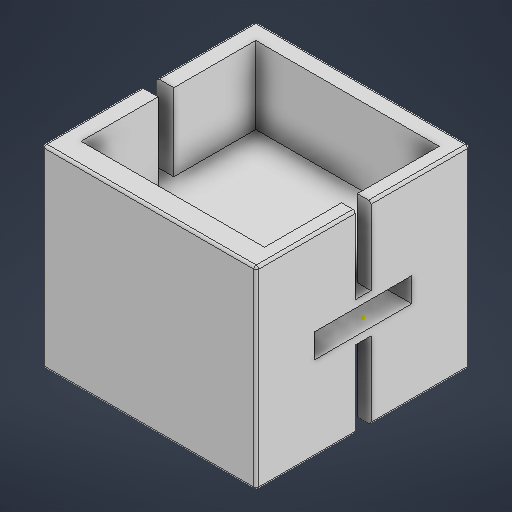
# Autodesk Inventor part: Base_Casing
Saved by Autodesk Inventor 2026.1 (Build 301233000, 233)
## iProperties
Created: 2025-09-05
Part Number: Base_Casing
Material: Generic
Document SubType Name: Modeling
Designer: usman
Density: 1 g/cm^3
Appearance: Default
Author: usman
Autodesk Inventor part; units mm, degrees
ref_plane "YZ Plane" through (0, 0, 0) normal (1, 0, 0) x (0, 1, 0)
ref_plane "XZ Plane" through (0, 0, 0) normal (0, 1, 0) x (-1, 0, 0)
ref_plane "XY Plane" through (0, 0, 0) normal (0, 0, 1) x (1, 0, 0)
sketch "Sketch1" plane through (0, 0, 0) normal (1, 0, 0) x (0, 1, 0)
  line L0 (-39.75, 43.9) -> (39.75, 43.9)
  line L1 (39.75, 43.9) -> (39.75, -43.9)
  line L2 (39.75, -43.9) -> (-39.75, -43.9)
  line L3 (-39.75, -43.9) -> (-39.75, 43.9)
  line L4 (-39.75, 43.9) -> (39.75, -43.9) construction
  line L5 (39.75, 43.9) -> (-39.75, -43.9) construction
  point P0 (0, 0)
  dimension "d0" = 79.5
  dimension "d1" = 87.8
  constraints: 12 end point, 2 midpoint, 2 parallel, 1 horizontal, 1 perpendicular
  measures "d0" distance of L1.end L2.end
  measures "d1" distance of L0.end L1.end
extrude "Extrusion1" add sketch "Sketch1" along normal blind 88
sketch "Sketch2" plane through (88, 0, 0) normal (1, 0, 0) x (0, 0, -1)
  line L0 (-20, -5) -> (20, -5)
  line L1 (20, -5) -> (20, 5)
  line L2 (20, 5) -> (-20, 5)
  line L3 (-20, 5) -> (-20, -5)
  line L4 (-20, -5) -> (20, 5) construction
  line L5 (20, -5) -> (-20, 5) construction
  point P0 (0, 0)
  dimension "d4" = 10
  dimension "d5" = 40
  constraints: 12 end point, 2 midpoint, 2 parallel, 1 horizontal, 1 perpendicular
  measures "d4" distance of L0.end L1.end
  measures "d5" distance of L1.end L2.end
extrude "Extrusion2" cut sketch "Sketch2" against normal through all
sketch "Sketch3" plane through (88, 0, 0) normal (1, 0, 0) x (0, 0, -1)
  point P0 (0, 0)
sketch "Sketch4" plane through (0, 39.75, 43.9) normal (0, 1, 0) x (1, 0, 0)
  line L0 (82.3836, 9.0103) -> (7, 9.0103)
  line L1 (7, 9.0103) -> (7, 80.8)
  line L2 (7, 80.8) -> (82.3836, 80.8)
  line L3 (82.3836, 80.8) -> (82.3836, 9.0103)
  line L4 (82.3836, 9.0103) -> (7, 80.8) construction
  line L5 (7, 9.0103) -> (82.3836, 80.8) construction
  line L6 (0, 87.8) -> (0, 0) projected
  line L7 (0, 87.8) -> (88, 87.8) projected
  point P0 (0, 43.9)
  point P1 (44.6918, 44.9051)
  dimension "d8" = 7
  dimension "d9" = 7
  constraints: 12 end point, 2 midpoint, 2 parallel, 1 horizontal, 1 perpendicular
  measures "d8" distance between parallel lines of L6 L1
  measures "d9" distance between parallel lines of L7 L2
extrude "Extrusion3" cut sketch "Sketch4" against normal blind 31.7
mirror "Mirror1" about plane through (0, 0, 0) normal (0, 1, 0) of "Extrusion3"
sketch "Sketch5" plane through (0, 0, 0) normal (-1, 0, 0) x (0, 0, 1)
  line L0 (-43.9, 39.75) -> (43.9, 39.75) projected
  line L1 (-3.25, 8.05) -> (3.25, 8.05)
  line L2 (3.25, 8.05) -> (3.25, 39.75)
  line L3 (3.25, 39.75) -> (-3.25, 39.75)
  line L4 (-3.25, 39.75) -> (-3.25, 8.05)
  line L5 (-3.25, 8.05) -> (3.25, 39.75) construction
  line L6 (3.25, 8.05) -> (-3.25, 39.75) construction
  point P0 (0, 0)
  point P1 (0, 23.9)
  point P2 (-3.25, 39.75)
  dimension "d12" = 3.25
  dimension "d13" = 31.7
  constraints: 12 end point, 2 midpoint, 2 parallel, 1 horizontal, 1 perpendicular, 1 point on line
  measures "d12" distance from line of point (0, 23.9) L2
  measures "d13" distance of L1.end L2.end
extrude "Extrusion4" cut sketch "Sketch5" against normal through all
mirror "Mirror2" about plane through (0, 0, 0) normal (0, 1, 0) of "Extrusion4"
sketch "Sketch6" plane through (0, 0, 0) normal (-1, 0, 0) x (0, 0, 1)
  line L0 (-43.5136, 38.271) -> (-4.0193, 38.271) construction
  line L1 (-4.0193, 38.271) -> (-4.0193, 7.5144) construction
  line L2 (-4.0193, 7.5144) -> (-43.5136, 7.5144) construction
  line L3 (-43.5136, 7.5144) -> (-43.5136, 38.271) construction
  line L4 (-32.9155, 25.9076) -> (-32.9155, 32.0036)
  line L5 (-32.9155, 32.0036) -> (-31.9606, 32.0036)
  spline S0 degree 2 poles (-31.9606, 32.0036) (-31.1264, 32.0036) (-30.7394, 31.898) knots 0 0 0 1 1 1
  spline S1 degree 2 poles (-30.7394, 31.898) (-30.1967, 31.7523) (-29.5484, 30.9633) (-29.5484, 30.4306) knots 0 0 0 1 2 2 2
  spline S2 degree 2 poles (-29.5484, 30.4306) (-29.5484, 30.0788) (-29.8398, 29.5109) (-30.1715, 29.2647) knots 0 0 0 1 2 2 2
  spline S3 degree 2 poles (-30.1715, 29.2647) (-29.6137, 29.0033) (-29.1011, 28.2193) (-29.1011, 27.6866) knots 0 0 0 1 2 2 2
  spline S4 degree 2 poles (-29.1011, 27.6866) (-29.1011, 27.169) (-29.6338, 26.3247) (-30.468, 25.9076) (-31.2068, 25.9076) knots 0 0 0 1 2 3 3 3
  line L6 (-31.2068, 25.9076) -> (-32.9155, 25.9076)
  line L7 (-31.7546, 28.5762) -> (-31.7546, 27.0132)
  line L8 (-31.7546, 27.0132) -> (-31.4631, 27.0132)
  spline S5 degree 2 poles (-31.4631, 27.0132) (-30.7444, 27.0132) (-30.2419, 27.3801) (-30.2419, 27.7268) knots 0 0 0 1 2 2 2
  spline S6 degree 2 poles (-30.2419, 27.7268) (-30.2419, 28.1188) (-30.8299, 28.5762) (-31.5134, 28.5762) knots 0 0 0 1 2 2 2
  line L9 (-31.5134, 28.5762) -> (-31.7546, 28.5762)
  line L10 (-31.7546, 30.898) -> (-31.7546, 29.6114)
  line L11 (-31.7546, 29.6114) -> (-31.5033, 29.6114)
  spline S7 degree 2 poles (-31.5033, 29.6114) (-31.0812, 29.6114) (-30.6691, 29.9682) (-30.6691, 30.2748) knots 0 0 0 1 2 2 2
  spline S8 degree 2 poles (-30.6691, 30.2748) (-30.6691, 30.5612) (-31.056, 30.898) (-31.4581, 30.898) knots 0 0 0 1 2 2 2
  line L12 (-31.4581, 30.898) -> (-31.7546, 30.898)
  line L13 (-24.7892, 30.4155) -> (-23.6584, 30.4155)
  line L14 (-23.6584, 30.4155) -> (-23.6584, 25.9076)
  line L15 (-23.6584, 25.9076) -> (-24.7892, 25.9076)
  line L16 (-24.7892, 25.9076) -> (-24.7892, 26.385)
  spline S9 degree 2 poles (-24.7892, 26.385) (-25.1208, 26.0684) (-25.7842, 25.792) (-26.1762, 25.792) knots 0 0 0 1 2 2 2
  spline S10 degree 2 poles (-26.1762, 25.792) (-27.0456, 25.792) (-28.3221, 27.1489) (-28.3221, 28.154) knots 0 0 0 1 2 2 2
  spline S11 degree 2 poles (-28.3221, 28.154) (-28.3221, 29.1993) (-27.0909, 30.5311) (-26.2064, 30.5311) knots 0 0 0 1 2 2 2
  spline S12 degree 2 poles (-26.2064, 30.5311) (-25.8043, 30.5311) (-25.0907, 30.2245) (-24.7892, 29.918) knots 0 0 0 1 2 2 2
  line L17 (-24.7892, 29.918) -> (-24.7892, 30.4155)
  spline S13 degree 2 poles (-25.9802, 29.4858) (-26.5029, 29.4858) (-27.1964, 28.747) (-27.1964, 28.1641) knots 0 0 0 1 2 2 2
  spline S14 degree 2 poles (-27.1964, 28.1641) (-27.1964, 27.5811) (-26.4878, 26.8273) (-25.9752, 26.8273) knots 0 0 0 1 2 2 2
  spline S15 degree 2 poles (-25.9752, 26.8273) (-25.4425, 26.8273) (-24.7389, 27.571) (-24.7389, 28.1691) knots 0 0 0 1 2 2 2
  spline S16 degree 2 poles (-24.7389, 28.1691) (-24.7389, 28.7571) (-25.4425, 29.4858) (-25.9802, 29.4858) knots 0 0 0 1 2 2 2
  line L18 (-19.7586, 29.7823) -> (-20.4571, 29.0837)
  spline S17 degree 2 poles (-20.4571, 29.0837) (-20.8793, 29.5059) (-21.226, 29.5059) knots 0 0 0 1 1 1
  spline S18 degree 2 poles (-21.226, 29.5059) (-21.417, 29.5059) (-21.6331, 29.3451) (-21.6331, 29.2244) knots 0 0 0 1 2 2 2
  spline S19 degree 2 poles (-21.6331, 29.2244) (-21.6331, 29.134) (-21.4974, 28.9782) (-21.226, 28.8475) knots 0 0 0 1 2 2 2
  line L19 (-21.226, 28.8475) -> (-20.8139, 28.6415)
  spline S20 degree 2 poles (-20.8139, 28.6415) (-20.1606, 28.3198) (-19.6731, 27.6464) (-19.6731, 27.1941) knots 0 0 0 1 2 2 2
  spline S21 degree 2 poles (-19.6731, 27.1941) (-19.6731, 26.5961) (-20.5526, 25.792) (-21.2964, 25.792) knots 0 0 0 1 2 2 2
  spline S22 degree 2 poles (-21.2964, 25.792) (-22.2814, 25.792) (-22.8694, 26.5609) knots 0 0 0 1 1 1
  line L20 (-22.8694, 26.5609) -> (-22.1759, 27.3198)
  spline S23 degree 2 poles (-22.1759, 27.3198) (-21.9748, 27.0886) (-21.4421, 26.8021) (-21.2361, 26.8021) knots 0 0 0 1 2 2 2
  spline S24 degree 2 poles (-21.2361, 26.8021) (-21.0099, 26.8021) (-20.7386, 27.0182) (-20.7386, 27.1589) knots 0 0 0 1 2 2 2
  spline S25 degree 2 poles (-20.7386, 27.1589) (-20.7386, 27.4203) (-21.2311, 27.6665) knots 0 0 0 1 1 1
  line L21 (-21.2311, 27.6665) -> (-21.613, 27.8575)
  spline S26 degree 2 poles (-21.613, 27.8575) (-22.7036, 28.4103) (-22.7036, 29.2395) knots 0 0 0 1 1 1
  spline S27 degree 2 poles (-22.7036, 29.2395) (-22.7036, 29.7722) (-21.8794, 30.5311) (-21.2411, 30.5311) knots 0 0 0 1 2 2 2
  spline S28 degree 2 poles (-21.2411, 30.5311) (-20.7989, 30.5311) (-20.0249, 30.1441) (-19.7586, 29.7823) knots 0 0 0 1 2 2 2
  line L22 (-14.2656, 27.8374) -> (-17.8941, 27.8374)
  spline S29 degree 2 poles (-17.8941, 27.8374) (-17.8137, 27.3549) (-17.1302, 26.7871) (-16.6025, 26.7871) knots 0 0 0 1 2 2 2
  spline S30 degree 2 poles (-16.6025, 26.7871) (-15.9693, 26.7871) (-15.512, 27.2293) knots 0 0 0 1 1 1
  line L23 (-15.512, 27.2293) -> (-14.5621, 26.782)
  spline S31 degree 2 poles (-14.5621, 26.782) (-14.919, 26.2795) (-15.914, 25.792) (-16.5975, 25.792) knots 0 0 0 1 2 2 2
  spline S32 degree 2 poles (-16.5975, 25.792) (-17.6579, 25.792) (-18.9897, 27.1288) (-18.9897, 28.1389) knots 0 0 0 1 2 2 2
  spline S33 degree 2 poles (-18.9897, 28.1389) (-18.9897, 29.1692) (-17.6579, 30.5311) (-16.6578, 30.5311) knots 0 0 0 1 2 2 2
  spline S34 degree 2 poles (-16.6578, 30.5311) (-15.5924, 30.5311) (-14.2606, 29.1692) (-14.2606, 28.0535) knots 0 0 0 1 2 2 2
  line L24 (-14.2606, 28.0535) -> (-14.2656, 27.8374)
  spline S35 degree 2 poles (-15.3964, 28.7269) (-15.507, 29.1038) (-16.1653, 29.5712) (-16.6025, 29.5712) knots 0 0 0 1 2 2 2
  spline S36 degree 2 poles (-16.6025, 29.5712) (-17.0749, 29.5712) (-17.4317, 29.3099) knots 0 0 0 1 1 1
  spline S37 degree 2 poles (-17.4317, 29.3099) (-17.6529, 29.144) (-17.8438, 28.7269) knots 0 0 0 1 1 1
  line L25 (-17.8438, 28.7269) -> (-15.3964, 28.7269)
  line L26 (-38.4386, 21.6418) -> (-37.3128, 21.6418)
  line L27 (-37.3128, 21.6418) -> (-35.8956, 17.3901)
  line L28 (-35.8956, 17.3901) -> (-34.4684, 21.6418)
  line L29 (-34.4684, 21.6418) -> (-33.3427, 21.6418)
  line L30 (-33.3427, 21.6418) -> (-32.3225, 15.5458)
  line L31 (-32.3225, 15.5458) -> (-33.4432, 15.5458)
  line L32 (-33.4432, 15.5458) -> (-34.0915, 19.3953)
  line L33 (-34.0915, 19.3953) -> (-35.3881, 15.5458)
  line L34 (-35.3881, 15.5458) -> (-36.4133, 15.5458)
  line L35 (-36.4133, 15.5458) -> (-37.6948, 19.3953)
  line L36 (-37.6948, 19.3953) -> (-38.3632, 15.5458)
  line L37 (-38.3632, 15.5458) -> (-39.4939, 15.5458)
  line L38 (-39.4939, 15.5458) -> (-38.4386, 21.6418)
  line L39 (-28.1864, 20.0537) -> (-27.0557, 20.0537)
  line L40 (-27.0557, 20.0537) -> (-27.0557, 15.5458)
  line L41 (-27.0557, 15.5458) -> (-28.1864, 15.5458)
  line L42 (-28.1864, 15.5458) -> (-28.1864, 16.0232)
  spline S38 degree 2 poles (-28.1864, 16.0232) (-28.5181, 15.7066) (-29.1815, 15.4302) (-29.5735, 15.4302) knots 0 0 0 1 2 2 2
  spline S39 degree 2 poles (-29.5735, 15.4302) (-30.4429, 15.4302) (-31.7194, 16.7871) (-31.7194, 17.7922) knots 0 0 0 1 2 2 2
  spline S40 degree 2 poles (-31.7194, 17.7922) (-31.7194, 18.8375) (-30.4881, 20.1693) (-29.6036, 20.1693) knots 0 0 0 1 2 2 2
  spline S41 degree 2 poles (-29.6036, 20.1693) (-29.2016, 20.1693) (-28.488, 19.8627) (-28.1864, 19.5562) knots 0 0 0 1 2 2 2
  line L43 (-28.1864, 19.5562) -> (-28.1864, 20.0537)
  spline S42 degree 2 poles (-29.3775, 19.124) (-29.9001, 19.124) (-30.5937, 18.3852) (-30.5937, 17.8022) knots 0 0 0 1 2 2 2
  spline S43 degree 2 poles (-30.5937, 17.8022) (-30.5937, 17.2193) (-29.8851, 16.4654) (-29.3725, 16.4654) knots 0 0 0 1 2 2 2
  spline S44 degree 2 poles (-29.3725, 16.4654) (-28.8398, 16.4654) (-28.1362, 17.2092) (-28.1362, 17.8073) knots 0 0 0 1 2 2 2
  spline S45 degree 2 poles (-28.1362, 17.8073) (-28.1362, 18.3953) (-28.8398, 19.124) (-29.3775, 19.124) knots 0 0 0 1 2 2 2
  line L44 (-22.5829, 20.0537) -> (-21.4522, 20.0537)
  line L45 (-21.4522, 20.0537) -> (-21.4522, 16.1941)
  spline S46 degree 2 poles (-21.4522, 16.1941) (-21.4522, 15.0482) (-21.9145, 14.5105) knots 0 0 0 1 1 1
  spline S47 degree 2 poles (-21.9145, 14.5105) (-22.5277, 13.7818) (-23.774, 13.7818) knots 0 0 0 1 1 1
  spline S48 degree 2 poles (-23.774, 13.7818) (-24.4374, 13.7818) (-25.3369, 14.1135) (-25.9601, 14.7568) (-26.1109, 15.2141) knots 0 0 0 1 2 3 3 3
  line L46 (-26.1109, 15.2141) -> (-24.8645, 15.2141)
  spline S49 degree 2 poles (-24.8645, 15.2141) (-24.6987, 15.0231) (-24.176, 14.8321) (-23.8192, 14.8321) knots 0 0 0 1 2 2 2
  spline S50 degree 2 poles (-23.8192, 14.8321) (-23.3669, 14.8321) (-22.8091, 15.1136) (-22.5829, 15.5608) (-22.5829, 16.1086) knots 0 0 0 1 2 3 3 3
  spline S51 degree 2 poles (-22.5829, 16.1086) (-22.8794, 15.8071) (-23.5328, 15.5458) (-23.9499, 15.5458) knots 0 0 0 1 2 2 2
  spline S52 degree 2 poles (-23.9499, 15.5458) (-24.8545, 15.5458) (-26.1059, 16.8574) (-26.1059, 17.8575) knots 0 0 0 1 2 2 2
  spline S53 degree 2 poles (-26.1059, 17.8575) (-26.1059, 18.933) (-25.4425, 19.5813) knots 0 0 0 1 1 1
  spline S54 degree 2 poles (-25.4425, 19.5813) (-24.8444, 20.1693) (-24.0102, 20.1693) knots 0 0 0 1 1 1
  spline S55 degree 2 poles (-24.0102, 20.1693) (-23.6232, 20.1693) (-22.9297, 19.8828) (-22.5829, 19.5562) knots 0 0 0 1 2 2 2
  line L47 (-22.5829, 19.5562) -> (-22.5829, 20.0537)
  spline S56 degree 2 poles (-23.7489, 19.1139) (-24.2866, 19.1139) (-24.9801, 18.3953) (-24.9801, 17.8525) knots 0 0 0 1 2 2 2
  spline S57 degree 2 poles (-24.9801, 17.8525) (-24.9801, 17.2896) (-24.2665, 16.571) (-23.7288, 16.571) knots 0 0 0 1 2 2 2
  spline S58 degree 2 poles (-23.7288, 16.571) (-23.2061, 16.571) (-22.5226, 17.2746) (-22.5226, 17.8475) knots 0 0 0 1 2 2 2
  spline S59 degree 2 poles (-22.5226, 17.8475) (-22.5226, 18.4103) (-23.2111, 19.1139) (-23.7489, 19.1139) knots 0 0 0 1 2 2 2
  line L48 (-20.3064, 20.0537) -> (-19.1756, 20.0537)
  line L49 (-19.1756, 20.0537) -> (-19.1756, 19.5913)
  spline S60 degree 2 poles (-19.1756, 19.5913) (-18.7886, 19.918) (-18.1655, 20.1693) (-17.8388, 20.1693) knots 0 0 0 1 2 2 2
  spline S61 degree 2 poles (-17.8388, 20.1693) (-17.1654, 20.1693) (-16.698, 19.7019) knots 0 0 0 1 1 1
  spline S62 degree 2 poles (-16.698, 19.7019) (-16.306, 19.3049) (-16.306, 18.5259) knots 0 0 0 1 1 1
  line L50 (-16.306, 18.5259) -> (-16.306, 15.5458)
  line L51 (-16.306, 15.5458) -> (-17.4267, 15.5458)
  line L52 (-17.4267, 15.5458) -> (-17.4267, 17.5208)
  spline S63 degree 2 poles (-17.4267, 17.5208) (-17.4267, 18.3249) (-17.5725, 18.8576) (-17.9293, 19.134) (-18.1956, 19.134) knots 0 0 0 1 2 3 3 3
  spline S64 degree 2 poles (-18.1956, 19.134) (-18.5374, 19.134) (-19.0299, 18.6767) (-19.1254, 18.2696) knots 0 0 0 1 2 2 2
  spline S65 degree 2 poles (-19.1254, 18.2696) (-19.1756, 18.0585) (-19.1756, 17.355) knots 0 0 0 1 1 1
  line L53 (-19.1756, 17.355) -> (-19.1756, 15.5458)
  line L54 (-19.1756, 15.5458) -> (-20.3064, 15.5458)
  line L55 (-20.3064, 15.5458) -> (-20.3064, 20.0537)
  line L56 (-10.6975, 17.4756) -> (-14.3259, 17.4756)
  spline S66 degree 2 poles (-14.3259, 17.4756) (-14.2455, 16.9931) (-13.5621, 16.4252) (-13.0344, 16.4252) knots 0 0 0 1 2 2 2
  spline S67 degree 2 poles (-13.0344, 16.4252) (-12.4012, 16.4252) (-11.9438, 16.8675) knots 0 0 0 1 1 1
  line L57 (-11.9438, 16.8675) -> (-10.994, 16.4202)
  spline S68 degree 2 poles (-10.994, 16.4202) (-11.3508, 15.9177) (-12.3459, 15.4302) (-13.0294, 15.4302) knots 0 0 0 1 2 2 2
  spline S69 degree 2 poles (-13.0294, 15.4302) (-14.0897, 15.4302) (-15.4215, 16.767) (-15.4215, 17.7771) knots 0 0 0 1 2 2 2
  spline S70 degree 2 poles (-15.4215, 17.7771) (-15.4215, 18.8074) (-14.0897, 20.1693) (-13.0897, 20.1693) knots 0 0 0 1 2 2 2
  spline S71 degree 2 poles (-13.0897, 20.1693) (-12.0242, 20.1693) (-10.6925, 18.8074) (-10.6925, 17.6917) knots 0 0 0 1 2 2 2
  line L58 (-10.6925, 17.6917) -> (-10.6975, 17.4756)
  spline S72 degree 2 poles (-11.8282, 18.3651) (-11.9388, 18.742) (-12.5972, 19.2094) (-13.0344, 19.2094) knots 0 0 0 1 2 2 2
  spline S73 degree 2 poles (-13.0344, 19.2094) (-13.5068, 19.2094) (-13.8636, 18.9481) knots 0 0 0 1 1 1
  spline S74 degree 2 poles (-13.8636, 18.9481) (-14.0847, 18.7822) (-14.2757, 18.3651) knots 0 0 0 1 1 1
  line L59 (-14.2757, 18.3651) -> (-11.8282, 18.3651)
  line L60 (-9.6421, 21.7172) -> (-8.5114, 21.7172)
  line L61 (-8.5114, 21.7172) -> (-8.5114, 20.0537)
  line L62 (-8.5114, 20.0537) -> (-7.838, 20.0537)
  line L63 (-7.838, 20.0537) -> (-7.838, 19.0787)
  line L64 (-7.838, 19.0787) -> (-8.5114, 19.0787)
  line L65 (-8.5114, 19.0787) -> (-8.5114, 15.5458)
  line L66 (-8.5114, 15.5458) -> (-9.6421, 15.5458)
  line L67 (-9.6421, 15.5458) -> (-9.6421, 19.0787)
  line L68 (-9.6421, 19.0787) -> (-10.2201, 19.0787)
  line L69 (-10.2201, 19.0787) -> (-10.2201, 20.0537)
  line L70 (-10.2201, 20.0537) -> (-9.6421, 20.0537)
  line L71 (-9.6421, 20.0537) -> (-9.6421, 21.7172)
  point P0 (0, 0)
  dimension "d0" = 79.5
  dimension "d1" = 87.8
  constraints: 2 other
sketch "Sketch7" plane through (0, 0, 0) normal (-1, 0, 0) x (0, 0, 1)
  line L0 (5.4174, 37.9215) -> (42.8146, 37.9215) construction
  line L1 (42.8146, 37.9215) -> (42.8146, 6.8154) construction
  line L2 (42.8146, 6.8154) -> (5.4174, 6.8154) construction
  line L3 (5.4174, 6.8154) -> (5.4174, 37.9215) construction
  line L4 (-40.9304, -8.5629) -> (-3.951, -8.5629) construction
  line L5 (-3.951, -8.5629) -> (-3.951, -37.9215) construction
  line L6 (-3.951, -37.9215) -> (-40.9304, -37.9215) construction
  line L7 (-40.9304, -37.9215) -> (-40.9304, -8.5629) construction
  line L8 (16.0675, 25.0873) -> (15.2584, 24.3133)
  spline S0 degree 2 poles (15.2584, 24.3133) (14.4292, 25.1878) (13.3939, 25.1878) knots 0 0 0 1 1 1
  spline S1 degree 2 poles (13.3939, 25.1878) (12.5195, 25.1878) (11.3234, 23.9967) (11.3234, 23.1223) knots 0 0 0 1 2 2 2
  spline S2 degree 2 poles (11.3234, 23.1223) (11.3234, 22.5142) (11.8511, 21.5694) (12.821, 21.0316) (13.414, 21.0316) knots 0 0 0 1 2 3 3 3
  spline S3 degree 2 poles (13.414, 21.0316) (13.9166, 21.0316) (14.7559, 21.4085) (15.2584, 21.9061) knots 0 0 0 1 2 2 2
  line L9 (15.2584, 21.9061) -> (16.0424, 21.0869)
  spline S4 degree 2 poles (16.0424, 21.0869) (15.369, 20.4235) (14.1679, 19.916) (13.3939, 19.916) knots 0 0 0 1 2 2 2
  spline S5 degree 2 poles (13.3939, 19.916) (11.9717, 19.916) (10.1625, 21.7151) (10.1625, 23.1273) knots 0 0 0 1 2 2 2
  spline S6 degree 2 poles (10.1625, 23.1273) (10.1625, 24.0369) (10.9867, 25.4541) (12.5245, 26.3135) (13.409, 26.3135) knots 0 0 0 1 2 3 3 3
  spline S7 degree 2 poles (13.409, 26.3135) (14.1679, 26.3135) (15.56, 25.6752) (16.0675, 25.0873) knots 0 0 0 1 2 2 2
  line L10 (20.289, 24.5746) -> (21.4198, 24.5746)
  line L11 (21.4198, 24.5746) -> (21.4198, 20.0667)
  line L12 (21.4198, 20.0667) -> (20.289, 20.0667)
  line L13 (20.289, 20.0667) -> (20.289, 20.5442)
  spline S8 degree 2 poles (20.289, 20.5442) (19.9573, 20.2275) (19.2939, 19.9511) (18.9019, 19.9511) knots 0 0 0 1 2 2 2
  spline S9 degree 2 poles (18.9019, 19.9511) (18.0325, 19.9511) (16.756, 21.308) (16.756, 22.3131) knots 0 0 0 1 2 2 2
  spline S10 degree 2 poles (16.756, 22.3131) (16.756, 23.3585) (17.9873, 24.6902) (18.8718, 24.6902) knots 0 0 0 1 2 2 2
  spline S11 degree 2 poles (18.8718, 24.6902) (19.2738, 24.6902) (19.9875, 24.3837) (20.289, 24.0771) knots 0 0 0 1 2 2 2
  line L14 (20.289, 24.0771) -> (20.289, 24.5746)
  spline S12 degree 2 poles (19.0979, 23.6449) (18.5753, 23.6449) (17.8818, 22.9062) (17.8818, 22.3232) knots 0 0 0 1 2 2 2
  spline S13 degree 2 poles (17.8818, 22.3232) (17.8818, 21.7402) (18.5904, 20.9864) (19.103, 20.9864) knots 0 0 0 1 2 2 2
  spline S14 degree 2 poles (19.103, 20.9864) (19.6357, 20.9864) (20.3393, 21.7302) (20.3393, 22.3282) knots 0 0 0 1 2 2 2
  spline S15 degree 2 poles (20.3393, 22.3282) (20.3393, 22.9162) (19.6357, 23.6449) (19.0979, 23.6449) knots 0 0 0 1 2 2 2
  line L15 (25.3196, 23.9414) -> (24.621, 23.2429)
  spline S16 degree 2 poles (24.621, 23.2429) (24.1989, 23.665) (23.8521, 23.665) knots 0 0 0 1 1 1
  spline S17 degree 2 poles (23.8521, 23.665) (23.6612, 23.665) (23.4451, 23.5042) (23.4451, 23.3836) knots 0 0 0 1 2 2 2
  spline S18 degree 2 poles (23.4451, 23.3836) (23.4451, 23.2931) (23.5807, 23.1373) (23.8521, 23.0067) knots 0 0 0 1 2 2 2
  line L16 (23.8521, 23.0067) -> (24.2642, 22.8006)
  spline S19 degree 2 poles (24.2642, 22.8006) (24.9175, 22.479) (25.405, 21.8056) (25.405, 21.3533) knots 0 0 0 1 2 2 2
  spline S20 degree 2 poles (25.405, 21.3533) (25.405, 20.7552) (24.5255, 19.9511) (23.7818, 19.9511) knots 0 0 0 1 2 2 2
  spline S21 degree 2 poles (23.7818, 19.9511) (22.7968, 19.9511) (22.2088, 20.72) knots 0 0 0 1 1 1
  line L17 (22.2088, 20.72) -> (22.9023, 21.4789)
  spline S22 degree 2 poles (22.9023, 21.4789) (23.1033, 21.2477) (23.636, 20.9613) (23.8421, 20.9613) knots 0 0 0 1 2 2 2
  spline S23 degree 2 poles (23.8421, 20.9613) (24.0682, 20.9613) (24.3396, 21.1774) (24.3396, 21.3181) knots 0 0 0 1 2 2 2
  spline S24 degree 2 poles (24.3396, 21.3181) (24.3396, 21.5794) (23.8471, 21.8257) knots 0 0 0 1 1 1
  line L18 (23.8471, 21.8257) -> (23.4652, 22.0166)
  spline S25 degree 2 poles (23.4652, 22.0166) (22.3746, 22.5695) (22.3746, 23.3987) knots 0 0 0 1 1 1
  spline S26 degree 2 poles (22.3746, 23.3987) (22.3746, 23.9314) (23.1988, 24.6902) (23.837, 24.6902) knots 0 0 0 1 2 2 2
  spline S27 degree 2 poles (23.837, 24.6902) (24.2793, 24.6902) (25.0532, 24.3033) (25.3196, 23.9414) knots 0 0 0 1 2 2 2
  line L19 (26.1739, 24.5746) -> (27.3047, 24.5746)
  line L20 (27.3047, 24.5746) -> (27.3047, 20.0667)
  line L21 (27.3047, 20.0667) -> (26.1739, 20.0667)
  line L22 (26.1739, 20.0667) -> (26.1739, 24.5746)
  spline S28 degree 2 poles (26.7368, 26.4341) (27.0333, 26.4341) (27.4605, 26.0019) (27.4605, 25.6953) knots 0 0 0 1 2 2 2
  spline S29 degree 2 poles (27.4605, 25.6953) (27.4605, 25.3938) (27.0383, 24.9666) (26.7468, 24.9666) knots 0 0 0 1 2 2 2
  spline S30 degree 2 poles (26.7468, 24.9666) (26.4453, 24.9666) (26.0181, 25.4039) (26.0181, 25.7104) knots 0 0 0 1 2 2 2
  spline S31 degree 2 poles (26.0181, 25.7104) (26.0181, 26.012) (26.4403, 26.4341) (26.7368, 26.4341) knots 0 0 0 1 2 2 2
  line L23 (28.3349, 24.5746) -> (29.4657, 24.5746)
  line L24 (29.4657, 24.5746) -> (29.4657, 24.1123)
  spline S32 degree 2 poles (29.4657, 24.1123) (29.8526, 24.439) (30.4758, 24.6902) (30.8025, 24.6902) knots 0 0 0 1 2 2 2
  spline S33 degree 2 poles (30.8025, 24.6902) (31.4759, 24.6902) (31.9433, 24.2229) knots 0 0 0 1 1 1
  spline S34 degree 2 poles (31.9433, 24.2229) (32.3353, 23.8258) (32.3353, 23.0469) knots 0 0 0 1 1 1
  line L25 (32.3353, 23.0469) -> (32.3353, 20.0667)
  line L26 (32.3353, 20.0667) -> (31.2146, 20.0667)
  line L27 (31.2146, 20.0667) -> (31.2146, 22.0418)
  spline S35 degree 2 poles (31.2146, 22.0418) (31.2146, 22.8459) (31.0688, 23.3786) (30.712, 23.655) (30.4457, 23.655) knots 0 0 0 1 2 3 3 3
  spline S36 degree 2 poles (30.4457, 23.655) (30.1039, 23.655) (29.6114, 23.1976) (29.5159, 22.7906) knots 0 0 0 1 2 2 2
  spline S37 degree 2 poles (29.5159, 22.7906) (29.4657, 22.5795) (29.4657, 21.8759) knots 0 0 0 1 1 1
  line L28 (29.4657, 21.8759) -> (29.4657, 20.0667)
  line L29 (29.4657, 20.0667) -> (28.3349, 20.0667)
  line L30 (28.3349, 20.0667) -> (28.3349, 24.5746)
  line L31 (36.7578, 24.5746) -> (37.8885, 24.5746)
  line L32 (37.8885, 24.5746) -> (37.8885, 20.715)
  spline S38 degree 2 poles (37.8885, 20.715) (37.8885, 19.5692) (37.4261, 19.0315) knots 0 0 0 1 1 1
  spline S39 degree 2 poles (37.4261, 19.0315) (36.813, 18.3028) (35.5667, 18.3028) knots 0 0 0 1 1 1
  spline S40 degree 2 poles (35.5667, 18.3028) (34.9033, 18.3028) (34.0037, 18.6344) (33.3806, 19.2777) (33.2298, 19.735) knots 0 0 0 1 2 3 3 3
  line L33 (33.2298, 19.735) -> (34.4761, 19.735)
  spline S41 degree 2 poles (34.4761, 19.735) (34.642, 19.5441) (35.1646, 19.3531) (35.5215, 19.3531) knots 0 0 0 1 2 2 2
  spline S42 degree 2 poles (35.5215, 19.3531) (35.9738, 19.3531) (36.5316, 19.6345) (36.7578, 20.0818) (36.7578, 20.6296) knots 0 0 0 1 2 3 3 3
  spline S43 degree 2 poles (36.7578, 20.6296) (36.4612, 20.3281) (35.8079, 20.0667) (35.3908, 20.0667) knots 0 0 0 1 2 2 2
  spline S44 degree 2 poles (35.3908, 20.0667) (34.4862, 20.0667) (33.2348, 21.3784) (33.2348, 22.3785) knots 0 0 0 1 2 2 2
  spline S45 degree 2 poles (33.2348, 22.3785) (33.2348, 23.4539) (33.8982, 24.1022) knots 0 0 0 1 1 1
  spline S46 degree 2 poles (33.8982, 24.1022) (34.4963, 24.6902) (35.3305, 24.6902) knots 0 0 0 1 1 1
  spline S47 degree 2 poles (35.3305, 24.6902) (35.7175, 24.6902) (36.411, 24.4038) (36.7578, 24.0771) knots 0 0 0 1 2 2 2
  line L34 (36.7578, 24.0771) -> (36.7578, 24.5746)
  spline S48 degree 2 poles (35.5918, 23.6349) (35.0541, 23.6349) (34.3606, 22.9162) (34.3606, 22.3735) knots 0 0 0 1 2 2 2
  spline S49 degree 2 poles (34.3606, 22.3735) (34.3606, 21.8106) (35.0742, 21.0919) (35.6119, 21.0919) knots 0 0 0 1 2 2 2
  spline S50 degree 2 poles (35.6119, 21.0919) (36.1346, 21.0919) (36.8181, 21.7955) (36.8181, 22.3684) knots 0 0 0 1 2 2 2
  spline S51 degree 2 poles (36.8181, 22.3684) (36.8181, 22.9313) (36.1296, 23.6349) (35.5918, 23.6349) knots 0 0 0 1 2 2 2
  line L35 (-39.6658, -20.1942) -> (-38.4848, -20.1942)
  line L36 (-38.4848, -20.1942) -> (-36.1429, -26.2902)
  line L37 (-36.1429, -26.2902) -> (-37.349, -26.2902)
  line L38 (-37.349, -26.2902) -> (-37.8265, -25.0338)
  line L39 (-37.8265, -25.0338) -> (-40.3141, -25.0338)
  line L40 (-40.3141, -25.0338) -> (-40.8066, -26.2902)
  line L41 (-40.8066, -26.2902) -> (-42.0128, -26.2902)
  line L42 (-42.0128, -26.2902) -> (-39.6658, -20.1942)
  line L43 (-39.0678, -21.8124) -> (-39.887, -23.9031)
  line L44 (-39.887, -23.9031) -> (-38.2587, -23.9031)
  line L45 (-38.2587, -23.9031) -> (-39.0678, -21.8124)
  spline S52 degree 2 poles (-33.5849, -20.0434) (-32.9165, -20.0434) (-31.9516, -20.6968) (-31.4239, -22.0436) (-31.4239, -23.2447) knots 0 0 0 1 2 3 3 3
  spline S53 degree 2 poles (-31.4239, -23.2447) (-31.4239, -24.4559) (-31.9566, -25.8077) (-32.8612, -26.441) (-33.5497, -26.441) knots 0 0 0 1 2 3 3 3
  spline S54 degree 2 poles (-33.5497, -26.441) (-34.2382, -26.441) (-35.173, -25.8027) (-35.7057, -24.5011) (-35.7057, -23.3) knots 0 0 0 1 2 3 3 3
  spline S55 degree 2 poles (-35.7057, -23.3) (-35.7057, -21.6265) (-35.1881, -20.8726) knots 0 0 0 1 1 1
  spline S56 degree 2 poles (-35.1881, -20.8726) (-34.6101, -20.0434) (-33.5849, -20.0434) knots 0 0 0 1 1 1
  spline S57 degree 2 poles (-33.5547, -21.144) (-33.8513, -21.144) (-34.3036, -21.5209) (-34.5448, -22.4406) (-34.5448, -23.3251) knots 0 0 0 1 2 3 3 3
  spline S58 degree 2 poles (-34.5448, -23.3251) (-34.5448, -24.481) (-33.997, -25.3655) (-33.5547, -25.3655) knots 0 0 0 1 2 2 2
  spline S59 degree 2 poles (-33.5547, -25.3655) (-33.1326, -25.3655) (-32.8864, -24.9484) knots 0 0 0 1 1 1
  spline S60 degree 2 poles (-32.8864, -24.9484) (-32.5848, -24.4408) (-32.5848, -23.2548) knots 0 0 0 1 1 1
  spline S61 degree 2 poles (-32.5848, -23.2548) (-32.5848, -22.0537) (-33.1276, -21.144) (-33.5547, -21.144) knots 0 0 0 1 2 2 2
  line L46 (-28.7302, -20.0434) -> (-27.7452, -20.5359)
  line L47 (-27.7452, -20.5359) -> (-28.8056, -22.6115)
  spline S62 degree 2 poles (-28.8056, -22.6115) (-28.0317, -22.6115) (-26.9461, -23.7221) (-26.9461, -24.5413) knots 0 0 0 1 2 2 2
  spline S63 degree 2 poles (-26.9461, -24.5413) (-26.9461, -25.3353) (-28.0618, -26.441) (-28.8458, -26.441) knots 0 0 0 1 2 2 2
  spline S64 degree 2 poles (-28.8458, -26.441) (-29.675, -26.441) (-30.7706, -25.2951) (-30.7706, -24.5564) knots 0 0 0 1 2 2 2
  spline S65 degree 2 poles (-30.7706, -24.5564) (-30.7706, -24.2749) (-30.5997, -23.7071) (-30.2932, -23.114) knots 0 0 0 1 2 2 2
  line L48 (-30.2932, -23.114) -> (-28.7302, -20.0434)
  spline S66 degree 2 poles (-28.8709, -23.7121) (-29.1976, -23.7121) (-29.6348, -24.1795) (-29.6348, -24.5262) knots 0 0 0 1 2 2 2
  spline S67 degree 2 poles (-29.6348, -24.5262) (-29.6348, -24.878) (-29.1775, -25.3554) (-28.8709, -25.3554) knots 0 0 0 1 2 2 2
  spline S68 degree 2 poles (-28.8709, -25.3554) (-28.5443, -25.3554) (-28.0819, -24.8881) (-28.0819, -24.5262) knots 0 0 0 1 2 2 2
  spline S69 degree 2 poles (-28.0819, -24.5262) (-28.0819, -24.1795) (-28.5342, -23.7121) (-28.8709, -23.7121) knots 0 0 0 1 2 2 2
  line L49 (-23.6142, -20.0434) -> (-22.4633, -20.0434)
  line L50 (-22.4633, -20.0434) -> (-22.4633, -23.9634)
  line L51 (-22.4633, -23.9634) -> (-21.9206, -23.9634)
  line L52 (-21.9206, -23.9634) -> (-21.9206, -25.0388)
  line L53 (-21.9206, -25.0388) -> (-22.4633, -25.0388)
  line L54 (-22.4633, -25.0388) -> (-22.4633, -26.2902)
  line L55 (-22.4633, -26.2902) -> (-23.5991, -26.2902)
  line L56 (-23.5991, -26.2902) -> (-23.5991, -25.0388)
  line L57 (-23.5991, -25.0388) -> (-26.2576, -25.0388)
  line L58 (-26.2576, -25.0388) -> (-26.2576, -23.9634)
  line L59 (-26.2576, -23.9634) -> (-23.6142, -20.0434)
  line L60 (-23.5991, -23.9634) -> (-23.5991, -21.923)
  line L61 (-23.5991, -21.923) -> (-24.9912, -23.9634)
  line L62 (-24.9912, -23.9634) -> (-23.5991, -23.9634)
  line L63 (-20.2622, -20.1942) -> (-17.4076, -20.1942)
  line L64 (-17.4076, -20.1942) -> (-17.4076, -21.2697)
  line L65 (-17.4076, -21.2697) -> (-19.3978, -21.2697)
  line L66 (-19.3978, -21.2697) -> (-19.644, -22.3753)
  spline S70 degree 2 poles (-19.644, -22.3753) (-19.5385, -22.3451) (-19.3425, -22.315) (-19.252, -22.315) knots 0 0 0 1 2 2 2
  spline S71 degree 2 poles (-19.252, -22.315) (-18.4228, -22.315) (-17.3222, -23.4457) (-17.3222, -24.3302) knots 0 0 0 1 2 2 2
  spline S72 degree 2 poles (-17.3222, -24.3302) (-17.3222, -25.2198) (-18.5384, -26.441) (-19.4078, -26.441) knots 0 0 0 1 2 2 2
  spline S73 degree 2 poles (-19.4078, -26.441) (-20.1868, -26.441) (-21.3024, -25.5565) (-21.4783, -24.7876) knots 0 0 0 1 2 2 2
  line L67 (-21.4783, -24.7876) -> (-20.2622, -24.7876)
  spline S74 degree 2 poles (-20.2622, -24.7876) (-20.1214, -25.074) (-19.6591, -25.3655) (-19.3827, -25.3655) knots 0 0 0 1 2 2 2
  spline S75 degree 2 poles (-19.3827, -25.3655) (-18.9957, -25.3655) (-18.458, -24.8127) (-18.458, -24.3755) knots 0 0 0 1 2 2 2
  spline S76 degree 2 poles (-18.458, -24.3755) (-18.458, -23.9533) (-18.9605, -23.4106) (-19.3173, -23.4106) knots 0 0 0 1 2 2 2
  spline S77 degree 2 poles (-19.3173, -23.4106) (-19.5083, -23.4106) (-19.8752, -23.6015) (-20.0511, -23.7925) knots 0 0 0 1 2 2 2
  line L68 (-20.0511, -23.7925) -> (-21.0009, -23.5814)
  line L69 (-21.0009, -23.5814) -> (-20.2622, -20.1942)
  spline S78 degree 2 poles (-14.5682, -20.0434) (-13.8998, -20.0434) (-12.9349, -20.6968) (-12.4072, -22.0436) (-12.4072, -23.2447) knots 0 0 0 1 2 3 3 3
  spline S79 degree 2 poles (-12.4072, -23.2447) (-12.4072, -24.4559) (-12.9399, -25.8077) (-13.8445, -26.441) (-14.533, -26.441) knots 0 0 0 1 2 3 3 3
  spline S80 degree 2 poles (-14.533, -26.441) (-15.2215, -26.441) (-16.1563, -25.8027) (-16.689, -24.5011) (-16.689, -23.3) knots 0 0 0 1 2 3 3 3
  spline S81 degree 2 poles (-16.689, -23.3) (-16.689, -21.6265) (-16.1713, -20.8726) knots 0 0 0 1 1 1
  spline S82 degree 2 poles (-16.1713, -20.8726) (-15.5934, -20.0434) (-14.5682, -20.0434) knots 0 0 0 1 1 1
  spline S83 degree 2 poles (-14.538, -21.144) (-14.8346, -21.144) (-15.2869, -21.5209) (-15.5281, -22.4406) (-15.5281, -23.3251) knots 0 0 0 1 2 3 3 3
  spline S84 degree 2 poles (-15.5281, -23.3251) (-15.5281, -24.481) (-14.9803, -25.3655) (-14.538, -25.3655) knots 0 0 0 1 2 2 2
  spline S85 degree 2 poles (-14.538, -25.3655) (-14.1159, -25.3655) (-13.8696, -24.9484) knots 0 0 0 1 1 1
  spline S86 degree 2 poles (-13.8696, -24.9484) (-13.5681, -24.4408) (-13.5681, -23.2548) knots 0 0 0 1 1 1
  spline S87 degree 2 poles (-13.5681, -23.2548) (-13.5681, -22.0537) (-14.1109, -21.144) (-14.538, -21.144) knots 0 0 0 1 2 2 2
  spline S88 degree 2 poles (-9.814, -20.0434) (-9.1456, -20.0434) (-8.1807, -20.6968) (-7.653, -22.0436) (-7.653, -23.2447) knots 0 0 0 1 2 3 3 3
  spline S89 degree 2 poles (-7.653, -23.2447) (-7.653, -24.4559) (-8.1857, -25.8077) (-9.0903, -26.441) (-9.7788, -26.441) knots 0 0 0 1 2 3 3 3
  spline S90 degree 2 poles (-9.7788, -26.441) (-10.4673, -26.441) (-11.4021, -25.8027) (-11.9348, -24.5011) (-11.9348, -23.3) knots 0 0 0 1 2 3 3 3
  spline S91 degree 2 poles (-11.9348, -23.3) (-11.9348, -21.6265) (-11.4172, -20.8726) knots 0 0 0 1 1 1
  spline S92 degree 2 poles (-11.4172, -20.8726) (-10.8392, -20.0434) (-9.814, -20.0434) knots 0 0 0 1 1 1
  spline S93 degree 2 poles (-9.7839, -21.144) (-10.0804, -21.144) (-10.5327, -21.5209) (-10.7739, -22.4406) (-10.7739, -23.3251) knots 0 0 0 1 2 3 3 3
  spline S94 degree 2 poles (-10.7739, -23.3251) (-10.7739, -24.481) (-10.2261, -25.3655) (-9.7839, -25.3655) knots 0 0 0 1 2 2 2
  spline S95 degree 2 poles (-9.7839, -25.3655) (-9.3617, -25.3655) (-9.1155, -24.9484) knots 0 0 0 1 1 1
  spline S96 degree 2 poles (-9.1155, -24.9484) (-8.8139, -24.4408) (-8.8139, -23.2548) knots 0 0 0 1 1 1
  spline S97 degree 2 poles (-8.8139, -23.2548) (-8.8139, -22.0537) (-9.3567, -21.144) (-9.7839, -21.144) knots 0 0 0 1 2 2 2
  line L70 (-6.0197, -20.1942) -> (-4.2859, -20.1942)
  line L71 (-4.2859, -20.1942) -> (-4.2859, -26.2902)
  line L72 (-4.2859, -26.2902) -> (-5.4368, -26.2902)
  line L73 (-5.4368, -26.2902) -> (-5.4368, -21.2847)
  line L74 (-5.4368, -21.2847) -> (-6.6931, -21.2847)
  line L75 (-6.6931, -21.2847) -> (-6.0197, -20.1942)
  point P0 (0, 0)
  dimension "d0" = 79.5
  dimension "d1" = 87.8
  constraints: 4 other
sketch "Sketch8" plane through (0, 0, 0) normal (-1, 0, 0) x (0, 0, 1)
  line L0 (5.4174, -8.5629) -> (42.1156, -8.5629) construction
  line L1 (42.1156, -8.5629) -> (42.1156, -38.6205) construction
  line L2 (42.1156, -38.6205) -> (5.4174, -38.6205) construction
  line L3 (5.4174, -38.6205) -> (5.4174, -8.5629) construction
  line L4 (6.4861, -17.3303) -> (5.3553, -17.3303)
  spline S0 degree 2 poles (5.3553, -17.3303) (5.4006, -16.3453) (6.5514, -15.2145) (7.451, -15.2145) knots 0 0 0 1 2 2 2
  spline S1 degree 2 poles (7.451, -15.2145) (8.0038, -15.2145) (8.8581, -15.6819) (9.3657, -16.5664) (9.3657, -17.0187) knots 0 0 0 1 2 3 3 3
  spline S2 degree 2 poles (9.3657, -17.0187) (9.3657, -17.5615) (8.7476, -18.8128) (7.9234, -19.6672) knots 0 0 0 1 2 2 2
  line L5 (7.9234, -19.6672) -> (7.2399, -20.3858)
  line L6 (7.2399, -20.3858) -> (9.416, -20.3858)
  line L7 (9.416, -20.3858) -> (9.416, -21.4613)
  line L8 (9.416, -21.4613) -> (5.1895, -21.4613)
  line L9 (5.1895, -21.4613) -> (5.1895, -20.9085)
  line L10 (5.1895, -20.9085) -> (7.0791, -18.9837)
  spline S3 degree 2 poles (7.0791, -18.9837) (7.7626, -18.2902) (8.2149, -17.4509) (8.2149, -17.1142) knots 0 0 0 1 2 2 2
  spline S4 degree 2 poles (8.2149, -17.1142) (8.2149, -16.7574) (7.7475, -16.3001) (7.3756, -16.3001) knots 0 0 0 1 2 2 2
  spline S5 degree 2 poles (7.3756, -16.3001) (7.0037, -16.3001) (6.5012, -16.8529) (6.4861, -17.3303) knots 0 0 0 1 2 2 2
  line L11 (12.5821, -15.2145) -> (13.7329, -15.2145)
  line L12 (13.7329, -15.2145) -> (13.7329, -19.1345)
  line L13 (13.7329, -19.1345) -> (14.2757, -19.1345)
  line L14 (14.2757, -19.1345) -> (14.2757, -20.2099)
  line L15 (14.2757, -20.2099) -> (13.7329, -20.2099)
  line L16 (13.7329, -20.2099) -> (13.7329, -21.4613)
  line L17 (13.7329, -21.4613) -> (12.5972, -21.4613)
  line L18 (12.5972, -21.4613) -> (12.5972, -20.2099)
  line L19 (12.5972, -20.2099) -> (9.9386, -20.2099)
  line L20 (9.9386, -20.2099) -> (9.9386, -19.1345)
  line L21 (9.9386, -19.1345) -> (12.5821, -15.2145)
  line L22 (12.5972, -19.1345) -> (12.5972, -17.0941)
  line L23 (12.5972, -17.0941) -> (11.2051, -19.1345)
  line L24 (11.2051, -19.1345) -> (12.5972, -19.1345)
  line L25 (15.2255, -15.2899) -> (16.3563, -15.2899)
  line L26 (16.3563, -15.2899) -> (16.3563, -16.9534)
  line L27 (16.3563, -16.9534) -> (17.0297, -16.9534)
  line L28 (17.0297, -16.9534) -> (17.0297, -17.9283)
  line L29 (17.0297, -17.9283) -> (16.3563, -17.9283)
  line L30 (16.3563, -17.9283) -> (16.3563, -21.4613)
  line L31 (16.3563, -21.4613) -> (15.2255, -21.4613)
  line L32 (15.2255, -21.4613) -> (15.2255, -17.9283)
  line L33 (15.2255, -17.9283) -> (14.6476, -17.9283)
  line L34 (14.6476, -17.9283) -> (14.6476, -16.9534)
  line L35 (14.6476, -16.9534) -> (15.2255, -16.9534)
  line L36 (15.2255, -16.9534) -> (15.2255, -15.2899)
  line L37 (17.6378, -15.2095) -> (18.7585, -15.2095)
  line L38 (18.7585, -15.2095) -> (18.7585, -17.4107)
  spline S6 degree 2 poles (18.7585, -17.4107) (19.0902, -17.1243) (19.7636, -16.8378) (20.1053, -16.8378) knots 0 0 0 1 2 2 2
  spline S7 degree 2 poles (20.1053, -16.8378) (20.7788, -16.8378) (21.2411, -17.3001) knots 0 0 0 1 1 1
  spline S8 degree 2 poles (21.2411, -17.3001) (21.6331, -17.7022) (21.6331, -18.4812) knots 0 0 0 1 1 1
  line L39 (21.6331, -18.4812) -> (21.6331, -21.4613)
  line L40 (21.6331, -21.4613) -> (20.5174, -21.4613)
  line L41 (20.5174, -21.4613) -> (20.5174, -19.4863)
  spline S9 degree 2 poles (20.5174, -19.4863) (20.5174, -18.7023) (20.3667, -18.1444) (20.0048, -17.8731) (19.7435, -17.8731) knots 0 0 0 1 2 3 3 3
  spline S10 degree 2 poles (19.7435, -17.8731) (19.3967, -17.8731) (18.9042, -18.3304) (18.8087, -18.7224) knots 0 0 0 1 2 2 2
  spline S11 degree 2 poles (18.8087, -18.7224) (18.7585, -18.9234) (18.7585, -19.6521) knots 0 0 0 1 1 1
  line L42 (18.7585, -19.6521) -> (18.7585, -21.4613)
  line L43 (18.7585, -21.4613) -> (17.6378, -21.4613)
  line L44 (17.6378, -21.4613) -> (17.6378, -15.2095)
  line L45 (28.4277, -16.1945) -> (27.5683, -16.9534)
  spline S12 degree 2 poles (27.5683, -16.9534) (27.116, -16.3252) (26.6486, -16.3252) knots 0 0 0 1 1 1
  spline S13 degree 2 poles (26.6486, -16.3252) (26.4225, -16.3252) (26.131, -16.5714) (26.131, -16.7222) knots 0 0 0 1 2 2 2
  spline S14 degree 2 poles (26.131, -16.7222) (26.131, -16.878) (26.2365, -17.0137) knots 0 0 0 1 1 1
  spline S15 degree 2 poles (26.2365, -17.0137) (26.3772, -17.1946) (27.0858, -17.7927) knots 0 0 0 1 1 1
  spline S16 degree 2 poles (27.0858, -17.7927) (27.7442, -18.3505) (27.8849, -18.4962) knots 0 0 0 1 1 1
  spline S17 degree 2 poles (27.8849, -18.4962) (28.2367, -18.853) (28.5332, -19.5013) (28.5332, -19.8833) knots 0 0 0 1 2 2 2
  spline S18 degree 2 poles (28.5332, -19.8833) (28.5332, -20.6371) (27.4979, -21.6121) (26.6637, -21.6121) knots 0 0 0 1 2 2 2
  spline S19 degree 2 poles (26.6637, -21.6121) (26.0154, -21.6121) (25.0455, -20.9738) (24.7037, -20.2904) knots 0 0 0 1 2 2 2
  line L46 (24.7037, -20.2904) -> (25.6787, -19.7024)
  spline S20 degree 2 poles (25.6787, -19.7024) (26.1159, -20.5115) (26.6888, -20.5115) knots 0 0 0 1 1 1
  spline S21 degree 2 poles (26.6888, -20.5115) (26.9853, -20.5115) (27.3924, -20.1647) (27.3924, -19.9335) knots 0 0 0 1 2 2 2
  spline S22 degree 2 poles (27.3924, -19.9335) (27.3924, -19.7275) (27.0858, -19.3154) (26.5632, -18.8882) knots 0 0 0 1 2 2 2
  spline S23 degree 2 poles (26.5632, -18.8882) (25.5681, -18.0741) (24.9902, -17.1946) (24.9902, -16.7574) knots 0 0 0 1 2 2 2
  spline S24 degree 2 poles (24.9902, -16.7574) (24.9902, -16.1191) (25.9551, -15.2145) (26.6637, -15.2145) knots 0 0 0 1 2 2 2
  spline S25 degree 2 poles (26.6637, -15.2145) (27.121, -15.2145) (27.9452, -15.6367) (28.4277, -16.1945) knots 0 0 0 1 2 2 2
  line L47 (34.0312, -19.5315) -> (30.4027, -19.5315)
  spline S26 degree 2 poles (30.4027, -19.5315) (30.4831, -20.0139) (31.1666, -20.5818) (31.6943, -20.5818) knots 0 0 0 1 2 2 2
  spline S27 degree 2 poles (31.6943, -20.5818) (32.3275, -20.5818) (32.7848, -20.1396) knots 0 0 0 1 1 1
  line L48 (32.7848, -20.1396) -> (33.7346, -20.5869)
  spline S28 degree 2 poles (33.7346, -20.5869) (33.3778, -21.0894) (32.3828, -21.5769) (31.6993, -21.5769) knots 0 0 0 1 2 2 2
  spline S29 degree 2 poles (31.6993, -21.5769) (30.6389, -21.5769) (29.3071, -20.2401) (29.3071, -19.23) knots 0 0 0 1 2 2 2
  spline S30 degree 2 poles (29.3071, -19.23) (29.3071, -18.1997) (30.6389, -16.8378) (31.639, -16.8378) knots 0 0 0 1 2 2 2
  spline S31 degree 2 poles (31.639, -16.8378) (32.7044, -16.8378) (34.0362, -18.1997) (34.0362, -19.3154) knots 0 0 0 1 2 2 2
  line L49 (34.0362, -19.3154) -> (34.0312, -19.5315)
  spline S32 degree 2 poles (32.9004, -18.642) (32.7898, -18.2651) (32.1315, -17.7977) (31.6943, -17.7977) knots 0 0 0 1 2 2 2
  spline S33 degree 2 poles (31.6943, -17.7977) (31.2219, -17.7977) (30.8651, -18.059) knots 0 0 0 1 1 1
  spline S34 degree 2 poles (30.8651, -18.059) (30.6439, -18.2249) (30.453, -18.642) knots 0 0 0 1 1 1
  line L50 (30.453, -18.642) -> (32.9004, -18.642)
  line L51 (36.0766, -16.9534) -> (36.0766, -17.4509)
  spline S35 degree 2 poles (36.0766, -17.4509) (36.3831, -17.1444) (37.0967, -16.8378) (37.4988, -16.8378) knots 0 0 0 1 2 2 2
  spline S36 degree 2 poles (37.4988, -16.8378) (38.3833, -16.8378) (39.6145, -18.1696) (39.6145, -19.2149) knots 0 0 0 1 2 2 2
  spline S37 degree 2 poles (39.6145, -19.2149) (39.6145, -20.22) (38.3381, -21.5769) (37.4686, -21.5769) knots 0 0 0 1 2 2 2
  spline S38 degree 2 poles (37.4686, -21.5769) (37.0766, -21.5769) (36.4082, -21.3005) (36.0766, -20.9839) knots 0 0 0 1 2 2 2
  line L52 (36.0766, -20.9839) -> (36.0766, -23.1097)
  line L53 (36.0766, -23.1097) -> (34.9508, -23.1097)
  line L54 (34.9508, -23.1097) -> (34.9508, -16.9534)
  line L55 (34.9508, -16.9534) -> (36.0766, -16.9534)
  spline S39 degree 2 poles (37.2626, -17.8831) (36.7299, -17.8831) (36.0263, -18.6118) (36.0263, -19.1998) knots 0 0 0 1 2 2 2
  spline S40 degree 2 poles (36.0263, -19.1998) (36.0263, -19.7978) (36.7299, -20.5416) (37.2626, -20.5416) knots 0 0 0 1 2 2 2
  spline S41 degree 2 poles (37.2626, -20.5416) (37.7802, -20.5416) (38.4888, -19.7878) (38.4888, -19.2048) knots 0 0 0 1 2 2 2
  spline S42 degree 2 poles (38.4888, -19.2048) (38.4888, -18.6219) (37.7953, -17.8831) (37.2626, -17.8831) knots 0 0 0 1 2 2 2
  line L56 (40.69, -15.2899) -> (41.8208, -15.2899)
  line L57 (41.8208, -15.2899) -> (41.8208, -16.9534)
  line L58 (41.8208, -16.9534) -> (42.4942, -16.9534)
  line L59 (42.4942, -16.9534) -> (42.4942, -17.9283)
  line L60 (42.4942, -17.9283) -> (41.8208, -17.9283)
  line L61 (41.8208, -17.9283) -> (41.8208, -21.4613)
  line L62 (41.8208, -21.4613) -> (40.69, -21.4613)
  line L63 (40.69, -21.4613) -> (40.69, -17.9283)
  line L64 (40.69, -17.9283) -> (40.1121, -17.9283)
  line L65 (40.1121, -17.9283) -> (40.1121, -16.9534)
  line L66 (40.1121, -16.9534) -> (40.69, -16.9534)
  line L67 (40.69, -16.9534) -> (40.69, -15.2899)
  line L68 (15.7356, -27.6921) -> (14.6049, -27.6921)
  spline S43 degree 2 poles (14.6049, -27.6921) (14.6501, -26.7071) (15.8009, -25.5764) (16.7005, -25.5764) knots 0 0 0 1 2 2 2
  spline S44 degree 2 poles (16.7005, -25.5764) (17.2533, -25.5764) (18.1077, -26.0437) (18.6153, -26.9282) (18.6153, -27.3805) knots 0 0 0 1 2 3 3 3
  spline S45 degree 2 poles (18.6153, -27.3805) (18.6153, -27.9233) (17.9971, -29.1747) (17.1729, -30.029) knots 0 0 0 1 2 2 2
  line L69 (17.1729, -30.029) -> (16.4895, -30.7477)
  line L70 (16.4895, -30.7477) -> (18.6655, -30.7477)
  line L71 (18.6655, -30.7477) -> (18.6655, -31.8231)
  line L72 (18.6655, -31.8231) -> (14.439, -31.8231)
  line L73 (14.439, -31.8231) -> (14.439, -31.2703)
  line L74 (14.439, -31.2703) -> (16.3286, -29.3455)
  spline S46 degree 2 poles (16.3286, -29.3455) (17.0121, -28.652) (17.4644, -27.8127) (17.4644, -27.476) knots 0 0 0 1 2 2 2
  spline S47 degree 2 poles (17.4644, -27.476) (17.4644, -27.1192) (16.997, -26.6619) (16.6251, -26.6619) knots 0 0 0 1 2 2 2
  spline S48 degree 2 poles (16.6251, -26.6619) (16.2532, -26.6619) (15.7507, -27.2147) (15.7356, -27.6921) knots 0 0 0 1 2 2 2
  spline S49 degree 2 poles (21.3693, -25.5764) (22.0377, -25.5764) (23.0026, -26.2297) (23.5303, -27.5765) (23.5303, -28.7776) knots 0 0 0 1 2 3 3 3
  spline S50 degree 2 poles (23.5303, -28.7776) (23.5303, -29.9888) (22.9975, -31.3407) (22.0929, -31.9739) (21.4044, -31.9739) knots 0 0 0 1 2 3 3 3
  spline S51 degree 2 poles (21.4044, -31.9739) (20.7159, -31.9739) (19.7812, -31.3356) (19.2485, -30.034) (19.2485, -28.8329) knots 0 0 0 1 2 3 3 3
  spline S52 degree 2 poles (19.2485, -28.8329) (19.2485, -27.1594) (19.7661, -26.4056) knots 0 0 0 1 1 1
  spline S53 degree 2 poles (19.7661, -26.4056) (20.3441, -25.5764) (21.3693, -25.5764) knots 0 0 0 1 1 1
  spline S54 degree 2 poles (21.3994, -26.677) (21.1029, -26.677) (20.6506, -27.0539) (20.4094, -27.9735) (20.4094, -28.858) knots 0 0 0 1 2 3 3 3
  spline S55 degree 2 poles (20.4094, -28.858) (20.4094, -30.0139) (20.9572, -30.8984) (21.3994, -30.8984) knots 0 0 0 1 2 2 2
  spline S56 degree 2 poles (21.3994, -30.8984) (21.8216, -30.8984) (22.0678, -30.4813) knots 0 0 0 1 1 1
  spline S57 degree 2 poles (22.0678, -30.4813) (22.3694, -29.9737) (22.3694, -28.7877) knots 0 0 0 1 1 1
  spline S58 degree 2 poles (22.3694, -28.7877) (22.3694, -27.5866) (21.8266, -26.677) (21.3994, -26.677) knots 0 0 0 1 2 2 2
  line L75 (25.244, -27.6921) -> (24.1132, -27.6921)
  spline S59 degree 2 poles (24.1132, -27.6921) (24.1585, -26.7071) (25.3093, -25.5764) (26.2089, -25.5764) knots 0 0 0 1 2 2 2
  spline S60 degree 2 poles (26.2089, -25.5764) (26.7617, -25.5764) (27.616, -26.0437) (28.1236, -26.9282) (28.1236, -27.3805) knots 0 0 0 1 2 3 3 3
  spline S61 degree 2 poles (28.1236, -27.3805) (28.1236, -27.9233) (27.5055, -29.1747) (26.6813, -30.029) knots 0 0 0 1 2 2 2
  line L76 (26.6813, -30.029) -> (25.9978, -30.7477)
  line L77 (25.9978, -30.7477) -> (28.1739, -30.7477)
  line L78 (28.1739, -30.7477) -> (28.1739, -31.8231)
  line L79 (28.1739, -31.8231) -> (23.9474, -31.8231)
  line L80 (23.9474, -31.8231) -> (23.9474, -31.2703)
  line L81 (23.9474, -31.2703) -> (25.837, -29.3455)
  spline S62 degree 2 poles (25.837, -29.3455) (26.5205, -28.652) (26.9728, -27.8127) (26.9728, -27.476) knots 0 0 0 1 2 2 2
  spline S63 degree 2 poles (26.9728, -27.476) (26.9728, -27.1192) (26.5054, -26.6619) (26.1335, -26.6619) knots 0 0 0 1 2 2 2
  spline S64 degree 2 poles (26.1335, -26.6619) (25.7616, -26.6619) (25.259, -27.2147) (25.244, -27.6921) knots 0 0 0 1 2 2 2
  line L82 (29.9378, -25.7271) -> (32.7924, -25.7271)
  line L83 (32.7924, -25.7271) -> (32.7924, -26.8026)
  line L84 (32.7924, -26.8026) -> (30.8022, -26.8026)
  line L85 (30.8022, -26.8026) -> (30.556, -27.9082)
  spline S65 degree 2 poles (30.556, -27.9082) (30.6615, -27.8781) (30.8575, -27.8479) (30.948, -27.8479) knots 0 0 0 1 2 2 2
  spline S66 degree 2 poles (30.948, -27.8479) (31.7772, -27.8479) (32.8778, -28.9787) (32.8778, -29.8632) knots 0 0 0 1 2 2 2
  spline S67 degree 2 poles (32.8778, -29.8632) (32.8778, -30.7527) (31.6616, -31.9739) (30.7922, -31.9739) knots 0 0 0 1 2 2 2
  spline S68 degree 2 poles (30.7922, -31.9739) (30.0132, -31.9739) (28.8975, -31.0894) (28.7217, -30.3205) knots 0 0 0 1 2 2 2
  line L86 (28.7217, -30.3205) -> (29.9378, -30.3205)
  spline S69 degree 2 poles (29.9378, -30.3205) (30.0786, -30.6069) (30.5409, -30.8984) (30.8173, -30.8984) knots 0 0 0 1 2 2 2
  spline S70 degree 2 poles (30.8173, -30.8984) (31.2043, -30.8984) (31.742, -30.3456) (31.742, -29.9084) knots 0 0 0 1 2 2 2
  spline S71 degree 2 poles (31.742, -29.9084) (31.742, -29.4862) (31.2395, -28.9435) (30.8826, -28.9435) knots 0 0 0 1 2 2 2
  spline S72 degree 2 poles (30.8826, -28.9435) (30.6917, -28.9435) (30.3248, -29.1344) (30.1489, -29.3254) knots 0 0 0 1 2 2 2
  line L87 (30.1489, -29.3254) -> (29.1991, -29.1143)
  line L88 (29.1991, -29.1143) -> (29.9378, -25.7271)
  point P0 (0, 0)
  dimension "d0" = 79.5
  dimension "d1" = 87.8
  constraints: 2 other
emboss "Emboss1" sketch "Sketch6" operation cut depth 1.5 direction (1, 0, 0)
emboss "Emboss2" sketch "Sketch7" operation cut depth 1.5 direction (1, 0, 0)
emboss "Emboss3" sketch "Sketch8" operation cut depth 1.5 direction (1, 0, 0)
fillet "Fillet1" radius 1 16 edges at (88, 0, 43.9) (0, 0, 43.9) (88, 0, -43.9) (0, 0, -43.9) (44, 39.75, -43.9) (88, 39.75, -23.575) (88, 39.75, 23.575) (44, 39.75, 43.9) (0, 39.75, 23.575) (0, 39.75, -23.575) (0, -39.75, -23.575) (0, -39.75, 23.575) (44, -39.75, 43.9) (88, -39.75, 23.575) (88, -39.75, -23.575) (44, -39.75, -43.9)
body "Solid1"
